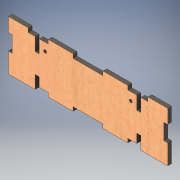
# Autodesk Inventor part: back
Saved by Autodesk Inventor 2019 (Build 230136000, 136)
## iProperties
Created: 2020-12-06
Part Number: back
Material: Дерево (береза)
Document SubType Name: Modeling
Designer: Professional
Density: 0.55 g/cm^3
Appearance: Береза — натуральный — полированный
Author: Professional
Autodesk Inventor part; units mm, degrees
ref_plane "YZ Plane" through (0, 0, 0) normal (1, 0, 0) x (0, 1, 0)
ref_plane "XZ Plane" through (0, 0, 0) normal (0, 1, 0) x (-1, 0, 0)
ref_plane "XY Plane" through (0, 0, 0) normal (0, 0, 1) x (1, 0, 0)
sketch "Эскиз1" plane through (0, 0, 0) normal (0, 0, 1) x (1, 0, 0)
  line L0 (0, 0) -> (-15, 0)
  line L1 (-15, 0) -> (-15, -4)
  line L2 (-15, -4) -> (-40, -4)
  line L3 (-40, -4) -> (-40, 0)
  line L4 (-40, 0) -> (-49, 0)
  line L5 (-49, 0) -> (-49, 9)
  line L6 (-49, 9) -> (-53, 9)
  line L7 (-53, 9) -> (-53, -4)
  line L8 (-53, -4) -> (-80, -4)
  line L9 (-80, 46) -> (-60, 46)
  line L10 (-60, 46) -> (-60, 42)
  line L11 (-60, 42) -> (-53, 42)
  line L12 (-53, 42) -> (-53, 29)
  line L13 (-53, 29) -> (-49, 29)
  line L14 (-49, 29) -> (-49, 42)
  line L15 (-49, 42) -> (-40, 42)
  line L16 (-40, 42) -> (-40, 46)
  line L17 (-40, 46) -> (-15, 46)
  line L18 (-15, 46) -> (-15, 42)
  line L19 (-15, 42) -> (0, 42)
  line L20 (0, 42) -> (0, 0)
  line L21 (0, 0) -> (15, 0)
  line L22 (15, 0) -> (15, -4)
  line L23 (15, -4) -> (40, -4)
  line L24 (40, -4) -> (40, 0)
  line L25 (40, 0) -> (49, 0)
  line L26 (49, 0) -> (49, 9)
  line L27 (49, 9) -> (53, 9)
  line L28 (53, 9) -> (53, -4)
  line L29 (53, -4) -> (80, -4)
  line L30 (80, 46) -> (60, 46)
  line L31 (60, 46) -> (60, 42)
  line L32 (60, 42) -> (53, 42)
  line L33 (53, 42) -> (53, 29)
  line L34 (53, 29) -> (49, 29)
  line L35 (49, 29) -> (49, 42)
  line L36 (49, 42) -> (40, 42)
  line L37 (40, 42) -> (40, 46)
  line L38 (40, 46) -> (15, 46)
  line L39 (15, 46) -> (15, 42)
  line L40 (15, 42) -> (0, 42)
  line L41 (-80, -4) -> (-80, 16)
  line L42 (-80, 16) -> (-76, 16)
  line L43 (-76, 16) -> (-76, 32)
  line L44 (-76, 32) -> (-80, 32)
  line L45 (-80, 32) -> (-80, 46)
  line L46 (80, -4) -> (80, 16)
  line L47 (76, 16) -> (76, 32)
  line L48 (76, 32) -> (80, 32)
  line L49 (80, 16) -> (76, 16)
  line L50 (80, 32) -> (80, 46)
  dimension "d0" = 4
  dimension "d1" = 30
  dimension "d2" = 25
  dimension "d3" = 9
  dimension "d4" = 20
  dimension "d5" = 13
  dimension "d6" = 17
  dimension "d9" = 25
  dimension "d12" = 20
  dimension "d13" = 27
  dimension "d14" = 16
  dimension "d15" = 14
  constraints: 102 end point, 24 symmetric about line, 22 point on line, 18 perpendicular, 4 equal length, 4 horizontal, 1 vertical, 1 vertical alignment
  measures "d0" distance of L0.end L1.end
  measures "d1" diameter of L1 L20
  measures "d2" distance of L1.end L2.end
  measures "d3" distance between parallel lines of L5 L3
  measures "d4" distance between parallel lines of L13 L6
  measures "d5" distance between parallel lines of L8 L6
  measures "d6" distance between parallel lines of L9 L13
  measures "d9" distance between parallel lines of L18 L16
  measures "d12" distance of L9.start L9.end
  measures "d13" distance of L7.end L8.end
  measures "d14" distance between parallel lines of L42 L44
  measures "d15" distance between parallel lines of L9 L44
extrude "Выдавливание1" add sketch "Эскиз1" along normal blind 4
sketch "Эскиз2" plane through (0, 0, 4) normal (0, 0, 1) x (1, 0, 0)
  circle A0 centre (-43, 34) radius 1.5
  line L0 (15, 42) -> (-15, 42) projected
  line L1 (0, 42) -> (0, 0)
  circle A1 centre (43, 34) radius 1.5
  dimension "d16" = 86
  dimension "d17" = 3
  dimension "d18" = 8
  constraints: 2 centre point, 2 end point, 1 midpoint, 1 symmetric about line, 1 vertical, 1 other
  measures "d16" distance of A1.centre A0.centre
  measures "d17" diameter of A0
  measures "d18" distance from line of A0.centre L0
extrude "Выдавливание2" cut sketch "Эскиз2" against normal through all
